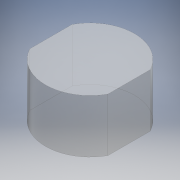
# Autodesk Inventor part: photodiode_cap
Saved by Autodesk Inventor 2016 (Build 200138000, 138)
## iProperties
Created: 2016-08-24
Part Number: photodiode_cap
Material: Polycarbonate, Clear
Document SubType Name: Modeling
Designer: rawrdong
Density: 1.2 g/cm^3
Appearance: Polycarbonate - Clear
Author: rawrdong
Autodesk Inventor part; units mm, degrees
ref_plane "YZ Plane" through (0, 0, 0) normal (1, 0, 0) x (0, 1, 0)
ref_plane "XZ Plane" through (0, 0, 0) normal (0, 1, 0) x (-1, 0, 0)
ref_plane "XY Plane" through (0, 0, 0) normal (0, 0, 1) x (1, 0, 0)
sketch "Sketch1" plane through (0, 0, 0) normal (0, 0, 1) x (1, 0, 0)
  circle A0 centre (0, 0) radius 1.25
  line L0 (-1.1, 0.5937) -> (-1.1, -0.5937)
  line L1 (1.1, 0.5937) -> (1.1, -0.5937)
  line L2 (0, 0) -> (0, 1.6774) construction
  dimension "d0" = 2.5
  dimension "d3" = 2.2
  constraints: 6 end point, 4 point on circle, 3 vertical, 1 centre point, 1 coincident, 1 other
  measures "d0" diameter of A0
  measures "d3" distance between parallel lines of L1 L0
extrude "Extrusion1" add sketch "Sketch1" against normal blind 1.5 contours L1 A0 L0
body "Solid1"
